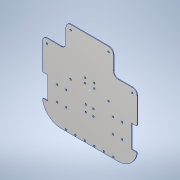
# Autodesk Inventor part: 台車土台
Saved by Autodesk Inventor 2020 (Build 240168000, 168)
## iProperties
Created: 2020-06-19
Part Number: 台車土台
Material: アルミニウム 6061
Document SubType Name: Modeling
Designer: jyajy
Density: 2.7 g/cm^3
Appearance: アルミニウム - フラット
Author: jyajy
Autodesk Inventor part; units mm, degrees
ref_plane "YZ Plane" through (0, 0, 0) normal (1, 0, 0) x (0, 1, 0)
ref_plane "XZ Plane" through (0, 0, 0) normal (0, 1, 0) x (-1, 0, 0)
ref_plane "XY Plane" through (0, 0, 0) normal (0, 0, 1) x (1, 0, 0)
sketch "スケッチ1" plane through (0, 0, 0) normal (0, 0, 1) x (1, 0, 0)
  line L0 (-100, -100) -> (100, -100)
  line L1 (100, -100) -> (100, 100)
  line L2 (100, 100) -> (-100, 100)
  line L3 (-100, 100) -> (-100, -100)
  line L4 (-100, -100) -> (100, 100) construction
  line L5 (100, -100) -> (-100, 100) construction
  point P0 (0, 0)
  dimension "d0" = 200
  dimension "d1" = 200
  constraints: 12 end point, 2 midpoint, 2 parallel, 1 horizontal, 1 perpendicular
  measures "d0" distance of L1.end L2.end
  measures "d1" distance of L2.end L0.start
extrude "押し出し1" add sketch "スケッチ1" along normal blind 1.5
fillet "フィレット1" radius 40 2 edges at (-100, -100, 0.75) (100, -100, 0.75)
sketch "スケッチ3" plane through (0, 0, 0) normal (0, 0, -1) x (-1, 0, 0)
  point P0 (0, 0)
sketch "スケッチ4" plane through (0, 0, 1.5) normal (0, 0, 1) x (1, 0, 0)
  line L0 (100, -60) -> (100, 100) projected
  line L1 (100, 100) -> (50, 100)
  line L2 (50, 100) -> (50, 50)
  line L3 (50, 50) -> (100, 50)
  line L4 (100, 50) -> (100, 100)
  line L5 (100, 100) -> (-100, 100) projected
  line L6 (-100, 100) -> (-50, 100)
  line L7 (-50, 100) -> (-50, 50)
  line L8 (-50, 50) -> (-100, 50)
  line L9 (-100, 50) -> (-100, 100)
  point P0 (0, 0)
  dimension "d13" = 50
  dimension "d14" = 50
  dimension "d15" = 50
  dimension "d16" = 50
  constraints: 16 end point, 4 parallel, 2 horizontal, 2 perpendicular
  measures "d13" distance of L0.end L1.end
  measures "d14" distance between parallel lines of L1 L3
  measures "d15" distance between parallel lines of L9 L7
  measures "d16" distance between parallel lines of L5 L8
extrude "押し出し2" cut sketch "スケッチ4" against normal through all
sketch "スケッチ5" plane through (0, 0, 1.5) normal (0, 0, 1) x (1, 0, 0)
  line L0 (-100, 50) -> (-100, -60) projected
  line L1 (-88, -64) -> (-100, -64)
  line L2 (-100, -64) -> (-100, -16)
  line L3 (-100, -16) -> (-88, -16)
  line L4 (-88, -16) -> (-88, -64)
  line L5 (-60, -100) -> (60, -100) projected
  line L6 (100, -60) -> (100, 50) projected
  line L7 (88, -64) -> (100, -64)
  line L8 (100, -64) -> (100, -16)
  line L9 (100, -16) -> (88, -16)
  line L10 (88, -16) -> (88, -64)
  point P0 (0, 0)
  dimension "d19" = 12
  dimension "d20" = 36
  dimension "d21" = 48
  dimension "d24" = 36
  dimension "d25" = 48
  dimension "d26" = 12
  constraints: 16 end point, 4 parallel, 2 horizontal, 2 perpendicular, 2 point on line
  measures "d19" distance between parallel lines of L4 L0
  measures "d20" distance between parallel lines of L1 L5
  measures "d21" distance between parallel lines of L1 L3
  measures "d24" distance between parallel lines of L7 L5
  measures "d25" distance between parallel lines of L7 L9
  measures "d26" distance between parallel lines of L6 L10
extrude "押し出し3" cut sketch "スケッチ5" against normal through all
fillet "フィレット2" radius 2 8 edges at (99.7995, -64, 0.75) (88, -64, 0.75) (100, -16, 0.75) (88, -16, 0.75) (-100, -16, 0.75) (-88, -16, 0.75) (-99.7995, -64, 0.75) (-88, -64, 0.75)
sketch "スケッチ6" plane through (0, 0, 1.5) normal (0, 0, 1) x (1, 0, 0)
  point P0 (0, 0)
fillet "フィレット3" radius 10 6 edges at (50, 100, 0.75) (50, 50, 0.75) (100, 50, 0.75) (-100, 50, 0.75) (-50, 50, 0.75) (-50, 100, 0.75)
sketch "スケッチ7" plane through (0, 0, 1.5) normal (0, 0, 1) x (1, 0, 0)
  line L0 (-100, 40) -> (-100, -14) projected
  line L1 (-60, 50) -> (-90, 50) projected
  line L2 (90, 50) -> (60, 50) projected
  line L3 (100, -14) -> (100, 40) projected
  line L4 (40, 100) -> (-40, 100) projected
  line L5 (50, 60) -> (50, 90) projected
  line L6 (-50, 90) -> (-50, 60) projected
  point P0 (0, 0)
  point P1 (-90, 40)
  point P2 (90, 40)
  point P3 (-40, 90)
  point P4 (40, 90)
  point P5 (40, 0)
  point P6 (-40, 0)
  dimension "d29" = 10
  dimension "d30" = 10
  dimension "d31" = 10
  dimension "d32" = 10
  dimension "d33" = 10
  dimension "d34" = 10
  dimension "d35" = 10
  dimension "d36" = 10
  dimension "d37" = 50
  dimension "d38" = 50
  constraints: 2 vertical alignment
  measures "d29" distance from line of point (-90, 40) L0
  measures "d30" distance from line of point (-90, 40) L1
  measures "d31" distance from line of point (90, 40) L2
  measures "d32" distance from line of point (90, 40) L3
  measures "d33" distance from line of point (40, 90) L4
  measures "d34" distance from line of point (40, 90) L5
  measures "d35" distance from line of point (-40, 90) L4
  measures "d36" distance from line of point (-40, 90) L6
  measures "d37" distance from line of point (40, 0) L2
  measures "d38" distance from line of L1 point (-40, 0)
hole "穴2" at (-90, 40, 1.5) at (90, 40, 1.5) at (-40, 90, 1.5) at (40, 90, 1.5) at (40, 0, 1.5) at (-40, 0, 1.5) direction (0, 0, -1) diameter 3.5 end through all
sketch "スケッチ8" plane through (0, 0, 1.5) normal (0, 0, 1) x (1, 0, 0)
  circle A0 centre (68.5, -55.9) radius 2.15 projected
  circle A1 centre (49.5, -55.9) radius 2.15 projected
  circle A2 centre (49.5, -24.1) radius 2.15 projected
  circle A3 centre (68.5, -24.1) radius 2.15 projected
  circle A4 centre (-49.5, -24.1) radius 2.15 projected
  circle A5 centre (-68.5, -24.1) radius 2.15 projected
  circle A6 centre (-49.5, -55.9) radius 2.15 projected
  circle A7 centre (-68.5, -55.9) radius 2.15 projected
  point P0 (0, 0)
hole "穴3" at (49.5, -55.9, 1.5) at (68.5, -55.9, 1.5) at (49.5, -24.1, 1.5) at (68.5, -24.1, 1.5) at (-49.5, -55.9, 1.5) at (-49.5, -24.1, 1.5) at (-68.5, -24.1, 1.5) at (-68.5, -55.9, 1.5) direction (0, 0, -1) diameter 3.5 end through all
sketch "スケッチ9" plane through (0, 0, 0) normal (0, 0, -1) x (-1, 0, 0)
  line L0 (0, 0) -> (0, -75.963)
  line L1 (60, -100) -> (-60, -100) projected
  point P0 (8, -44)
  point P1 (-8, -44)
  point P2 (8, -30)
  point P3 (-8, -30)
  dimension "d53" = 14
  dimension "d54" = 16
  dimension "d62" = 56
  constraints: 2 end point, 2 symmetric about line, 1 vertical, 1 vertical alignment
  measures "d53" distance of point (-8, -30) point (-8, -44)
  measures "d54" distance of point (-8, -44) point (8, -44)
  measures "d62" distance from line of point (-8, -44) L1
hole "穴4" at (-8, -44, 0) at (8, -44, 0) at (-8, -30, 0) at (8, -30, 0) direction (0, 0, 1) diameter 3.5 end through all
sketch "スケッチ10" plane through (0, 0, 0) normal (0, 0, -1) x (-1, 0, 0)
  line L0 (0, 0) -> (0, -140.1942)
  line L1 (60, -100) -> (-60, -100) projected
  point P0 (-10, -97)
  point P1 (10, -97)
  point P2 (-30, -97)
  point P3 (-50, -97)
  point P4 (30, -97)
  point P5 (50, -97)
  dimension "d63" = 10
  dimension "d64" = 3
  dimension "d65" = 20
  dimension "d66" = 20
  constraints: 3 symmetric about line, 2 end point, 2 horizontal alignment, 1 vertical
  measures "d63" distance from line of point (-10, -97) L0
  measures "d64" distance from line of point (-10, -97) L1
  measures "d65" distance of point (-30, -97) point (-10, -97)
  measures "d66" distance of point (-50, -97) point (-30, -97)
hole "穴5" at (10, -97, 0) at (-10, -97, 0) at (30, -97, 0) at (50, -97, 0) at (-30, -97, 0) at (-50, -97, 0) direction (0, 0, 1) diameter 3.5 end through all
sketch "スケッチ11" plane through (0, 0, 0) normal (0, 0, -1) x (-1, 0, 0)
  circle A0 centre (-9.7395, 8) radius 2.25 projected
  circle A1 centre (-9.7395, 18) radius 2.25 projected
  circle A2 centre (9.7395, 18) radius 2.25 projected
  circle A3 centre (9.7395, 8) radius 2.25 projected
  arc A4 (15, 20) -> (13, 22) centre (13, 20) ccw projected
  line L0 (14, 4) -> (-14, 4) projected
  arc A5 (-13, 22) -> (-15, 20) centre (-13, 20) ccw projected
  line L1 (-13, 22) -> (13, 22) projected
  line L2 (15, 20) -> (15, 3) projected
  arc A6 (15, 3) -> (14, 4) centre (14, 3) ccw projected
  arc A7 (-14, 4) -> (-15, 3) centre (-14, 3) ccw projected
  line L3 (-15, 3) -> (-15, 20) projected
  point P0 (0, 0)
  point P1 (15, 4)
  point P2 (-15, 4)
hole "穴6" at (9.7395, 8, 0) at (-9.7395, 8, 0) at (-9.7395, 18, 0) at (9.7395, 18, 0) direction (0, 0, 1) diameter 3.5 end through all
